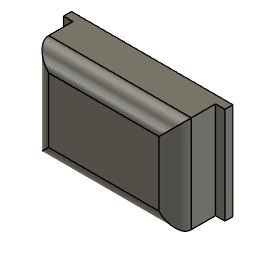
mds-0027 (Autodesk Fusion 360 archive; units mm, degrees)
design "Side-Button"
Autodesk Fusion 360 part; units mm, degrees
note: some values were not read from the file. Chosen so that the rebuilt part matches the saved one: which bodies a step acts on; which face or edge a step refers to. Set by a fixed rule: which sketch regions a step uses.
sketch "Sketch1" plane through (0, 0, 0) normal (0, 0, 1) x (1, 0, 0)
  line L0 (-30, 20) -> (-12.335, 20)
  line L1 (-12.335, 20) -> (-12.335, 8)
  line L2 (-12.335, 8) -> (-30, 8)
  line L3 (-30, 8) -> (-30, 20)
  dimension "d1" = 17.665
  dimension "d2" = 12
  constraint horizontal L0
  constraint vertical L1
  constraint horizontal L2
  constraint vertical L3
  measures "d1" distance of L0.start L0.end
  measures "d2" distance of L0.start L2.end
extrude "Extrude1" add sketch "Sketch1" along normal blind 6
fillet "Fillet1" radius 2 4 edges at (-21.1675, 20, 6) (-12.335, 14, 6) (-30, 14, 6) (-21.1675, 8, 6)
sketch "Sketch2" plane through (0, 0, 0) normal (0, 0, -1) x (-1, 0, 0)
  line L0 (12.335, 8) -> (30, 8)
  line L1 (30, 8) -> (30, 20)
  line L2 (30, 20) -> (12.335, 20)
  line L3 (12.335, 20) -> (12.335, 8)
  line L4 (11.1675, 20) -> (31.1675, 20)
  line L5 (11.1675, 8) -> (31.1675, 8)
  line L6 (31.1675, 20) -> (31.1675, 8)
  line L7 (11.1675, 8) -> (11.1675, 20)
  point P0 (21.1675, 20)
  point P1 (21.1675, 8)
  dimension "d7" = 20
  constraint midpoint L4 P0
  constraint coincident L2 P0
  constraint parallel L2 L4
  constraint midpoint L5 P1
  constraint coincident L0 P1
  constraint perpendicular L1 L5
  constraint perpendicular L5 L6
  constraint perpendicular L4 L7
  measures "d7" distance of L4.start L4.end
extrude "Extrude2" add sketch "Sketch2" against normal blind 1 contours L3 L4 L5 L7 | L1 L4 L5 L6

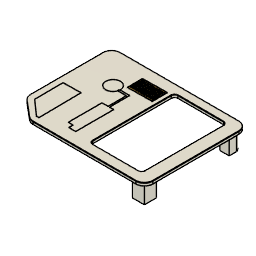
design "Lid" references "Main Casing"
Autodesk Fusion 360 part; units mm, degrees
other "Sketch2"
sketch "sketch 220" plane through (0, 0, 0) normal (0, 1, 0) x (1, 0, 0)
  line L0 (47.500001, 39.500001) -> (45.536455, 39.500001)
  line L1 (52.536455, 32.500001) -> (52.536455, 33)
  line L2 (45.536455, 39.500001) -> (-52.546208, 39.500001)
  line L3 (-59.546208, 32.500001) -> (-59.546208, -27.533953)
  line L4 (-39.426481, -45.554934) -> (45.536455, -45.554934)
  line L5 (52.536455, -38.554934) -> (52.536455, 32.500001)
  arc A0 (-52.546208, 39.500001) -> (-59.546208, 32.500001) centre (-52.546208, 32.500001) ccw
  arc A1 (45.536455, -45.554934) -> (52.536455, -38.554934) centre (45.536455, -38.554934) ccw
  line L6 (-57.048651, -32.893804) -> (-43.928925, -43.914786)
  arc A2 (-43.928925, -43.914786) -> (-39.426481, -45.554934) centre (-39.426481, -38.554934) ccw
  arc A3 (-59.546208, -27.533953) -> (-57.048651, -32.893804) centre (-52.546208, -27.533953) ccw
  line L7 (-57.046208, 32.500001) -> (-57.046208, -27.533953)
  arc A4 (-57.046208, -27.533953) -> (-55.440635, -30.979572) centre (-52.546208, -27.533953) ccw
  line L8 (-55.440635, -30.979572) -> (-42.320909, -42.000553)
  arc A5 (-42.320909, -42.000553) -> (-39.426481, -43.054934) centre (-39.426481, -38.554934) ccw
  line L9 (-39.426481, -43.054934) -> (45.536455, -43.054934)
  arc A6 (45.536455, -43.054934) -> (50.036455, -38.554934) centre (45.536455, -38.554934) ccw
  line L10 (50.036455, -38.554934) -> (50.036455, 32.500001)
  line L11 (45.536455, 37.000001) -> (-52.546208, 37.000001)
  arc A7 (-52.546208, 37.000001) -> (-57.046208, 32.500001) centre (-52.546208, 32.500001) ccw
  arc A8 (52.536455, 32.500001) -> (45.536455, 39.500001) centre (45.536455, 32.500001) ccw
  arc A9 (50.036455, 32.500001) -> (45.536455, 37.000001) centre (45.536455, 32.500001) ccw
extrude "Extrude1" add sketch "sketch 220" along normal blind 2 contours L2 L3 L4 L5 A0 A1 L6 A2 A3 A8 | L7 A4 L8 A5 L9 A6 L10 L11 A7 A9 picked at (-19.851987, 38.666667) picked at (-15.478745, 10.315022) makes body 1
sketch "Sketch2 (1)" plane through (0, 2, 0) normal (0, 1, 0) x (-1, 0, 0)
  arc A0 (59.546208, 27.533953) -> (57.048651, 32.893804) centre (52.546208, 27.533953) ccw
  line L0 (57.048651, 32.893804) -> (43.928925, 43.914786)
  arc A1 (43.928925, 43.914786) -> (39.426481, 45.554934) centre (39.426481, 38.554934) ccw
  line L1 (39.426481, 45.554934) -> (-45.536455, 45.554934)
  arc A2 (-45.536455, 45.554934) -> (-52.536455, 38.554934) centre (-45.536455, 38.554934) ccw
  line L2 (-52.536455, 38.554934) -> (-52.536455, -32.500001)
  line L3 (-45.536455, -39.500001) -> (52.546208, -39.500001)
  arc A3 (52.546208, -39.500001) -> (59.546208, -32.500001) centre (52.546208, -32.500001) ccw
  line L4 (59.546208, -32.500001) -> (59.546208, 27.533953)
  line L5 (39.853527, 5.449503) -> (39.426481, 40.606798)
  line L6 (39.426481, 40.606798) -> (41.485756, 40.631812)
  line L7 (41.485756, 40.631812) -> (54.299999, 29.299999)
  line L8 (54.299999, 29.299999) -> (54.499999, 5.7)
  line L9 (54.499999, 5.7) -> (39.853527, 5.449503)
  line L10 (4.205552, -17.763056) -> (24.5, -17.5)
  line L11 (24.5, -17.5) -> (24.662478, -30.03501)
  line L12 (24.662478, -30.03501) -> (4.288926, -30.299091)
  line L13 (4.288926, -30.299091) -> (4.205552, -17.763056)
  arc A4 (-52.536455, -32.500001) -> (-45.536455, -39.500001) centre (-45.536455, -32.500001) ccw
  constraint perpendicular L5 L6
  constraint perpendicular L10 L11
  constraint perpendicular L11 L12
extrude "Extrude2" add sketch "Sketch2 (1)" along normal blind 0.5 contours L5 L6 L7 L8 L9 | L10 L11 L12 L13 picked at (44.526669, 25.118767) picked at (11.052319, -26.032386) bodies 1
sketch "Sketch2" plane through (0, 2, 0) normal (0, 1, 0) x (-1, 0, 0)
  line L0 (54.499999, 5.7) -> (39.853527, 5.449503)
  line L1 (39.853527, 5.449503) -> (39.426481, 40.606798)
  line L2 (39.426481, 40.606798) -> (41.485756, 40.631812)
  line L3 (41.485756, 40.631812) -> (54.299999, 29.299999)
  line L4 (54.299999, 29.299999) -> (54.499999, 5.7)
  line L5 (4.288926, -30.299091) -> (4.205552, -17.763056)
  line L6 (4.205552, -17.763056) -> (24.5, -17.5)
  line L7 (24.5, -17.5) -> (24.662478, -30.03501)
  line L8 (24.662478, -30.03501) -> (4.288926, -30.299091)
  arc A0 (59.546208, 27.533953) -> (57.048651, 32.893804) centre (52.546208, 27.533953) ccw
  line L9 (57.048651, 32.893804) -> (43.928925, 43.914786)
  arc A1 (43.928925, 43.914786) -> (39.426481, 45.554934) centre (39.426481, 38.554934) ccw
  line L10 (39.426481, 45.554934) -> (-45.536455, 45.554934)
  arc A2 (-45.536455, 45.554934) -> (-52.536455, 38.554934) centre (-45.536455, 38.554934) ccw
  line L11 (-52.536455, 38.554934) -> (-52.536455, -32.500001)
  line L12 (-45.536455, -39.500001) -> (52.546208, -39.500001)
  arc A3 (52.546208, -39.500001) -> (59.546208, -32.500001) centre (52.546208, -32.500001) ccw
  line L13 (59.546208, -32.500001) -> (59.546208, 27.533953)
  line L14 (-42.294458, -30.655503) -> (3.504877, -30.655503)
  line L15 (3.504877, -30.655503) -> (3.504877, 35.741851)
  line L16 (3.504877, 35.741851) -> (-42.294458, 35.741851)
  line L17 (-42.294458, 35.741851) -> (-42.294458, -30.655503)
  line L18 (11, 17) -> (3.504877, 17)
  line L19 (3.504877, 17) -> (3.504877, 31.823372)
  line L20 (3.504877, 31.823372) -> (11, 31.823372)
  line L21 (11, 31.823372) -> (11, 17)
  line L22 (24, 4) -> (14.343, 4)
  line L23 (14.343, 4) -> (14.343, 31.823372)
  line L24 (14.343, 31.823372) -> (24, 31.823372)
  line L25 (24, 31.823372) -> (24, 4)
  line L26 (20.047669, 31.823372) -> (14.343, 31.823372)
  line L27 (14.343, 31.823372) -> (14.343, 35.373002)
  line L28 (14.343, 35.373002) -> (20.047669, 35.373002)
  line L29 (20.047669, 35.373002) -> (20.047669, 31.823372)
  line L30 (19, 4) -> (17.792239, 4)
  line L31 (17.792239, 4) -> (17.792239, -12.601724)
  line L32 (17.792239, -12.601724) -> (19, -12.601724)
  line L33 (19, -12.601724) -> (19, 4)
  line L34 (19, -12.601724) -> (26.334489, -12.601724)
  line L35 (26.334489, -12.601724) -> (26.334489, -11.113985)
  line L36 (26.334489, -11.113985) -> (19, -11.113985)
  line L37 (19, -11.113985) -> (19, -12.601724)
  circle A4 centre (31.789244, -12.921514) radius 6.052195
  arc A5 (-52.536455, -32.500001) -> (-45.536455, -39.500001) centre (-45.536455, -32.500001) ccw
  constraint horizontal L14
  constraint vertical L15
  constraint horizontal L16
  constraint vertical L17
  constraint horizontal L18
  constraint vertical L19
  constraint horizontal L20
  constraint vertical L21
  constraint horizontal L22
  constraint vertical L23
  constraint horizontal L24
  constraint vertical L25
  constraint horizontal L26
  constraint vertical L27
  constraint horizontal L28
  constraint vertical L29
  constraint horizontal L30
  constraint vertical L31
  constraint horizontal L32
  constraint vertical L33
  constraint coincident L22 L30.start
  constraint horizontal L34
  constraint vertical L35
  constraint horizontal L36
  constraint vertical L37
extrude "Extrude3" add sketch "Sketch2" along normal blind 0.5 separate body contours L14 L15 L16 L17 L19 | L15 L18 L19 L20 L21 | L22 L23 L24 L25 L26 L30 | L22 L30 L31 L32 L33 L37 | L33 L34 L36 L37 A4 | L24 L26 L27 L28 L29 | L34 L35 L36 A4 picked at (-27.028013, 7.362116) picked at (8.501626, 26.882248) picked at (17.394302, 22.548915) picked at (18.194826, -6.571903) picked at (21.264404, -11.938213) picked at (18.146112, 33.006582) picked at (33.983321, -12.514669) makes body 2 at (-33.99295, 2, -12.93937) makes body 2 at (-16.244556, 2, 23.732125) makes body 3 at (27.028013, 2, 7.362116)
sketch "Sketch3" plane through (0, 2, 0) normal (0, 1, 0) x (-1, 0, 0)
  line L0 (54.499999, 5.7) -> (39.853527, 5.449503)
  line L1 (39.853527, 5.449503) -> (39.426481, 40.606798)
  line L2 (39.426481, 40.606798) -> (41.485756, 40.631812)
  line L3 (41.485756, 40.631812) -> (54.299999, 29.299999)
  line L4 (54.299999, 29.299999) -> (54.499999, 5.7)
  line L5 (4.288926, -30.299091) -> (4.205552, -17.763056)
  line L6 (4.205552, -17.763056) -> (24.5, -17.5)
  line L7 (24.5, -17.5) -> (24.662478, -30.03501)
  line L8 (24.662478, -30.03501) -> (4.288926, -30.299091)
  arc A0 (59.546208, 27.533953) -> (57.048651, 32.893804) centre (52.546208, 27.533953) ccw
  line L9 (57.048651, 32.893804) -> (43.928925, 43.914786)
  arc A1 (43.928925, 43.914786) -> (39.426481, 45.554934) centre (39.426481, 38.554934) ccw
  line L10 (39.426481, 45.554934) -> (-45.536455, 45.554934)
  arc A2 (-45.536455, 45.554934) -> (-52.536455, 38.554934) centre (-45.536455, 38.554934) ccw
  line L11 (-52.536455, 38.554934) -> (-52.536455, -32.500001)
  line L12 (-45.536455, -39.500001) -> (52.546208, -39.500001)
  arc A3 (52.546208, -39.500001) -> (59.546208, -32.500001) centre (52.546208, -32.500001) ccw
  line L13 (59.546208, -32.500001) -> (59.546208, 27.533953)
  line L14 (3.505741, -0.818006) -> (21.505741, -0.818006)
  line L15 (21.505741, -0.818006) -> (21.505741, 9)
  line L16 (21.505741, 9) -> (3.505741, 9)
  line L17 (3.505741, 9) -> (3.505741, -0.818006)
  circle A4 centre (26.7, 3.4) radius 7.710383
  circle A5 centre (26.7, 3.4) radius 3.809172
  line L18 (26.255748, -0.383177) -> (26.255748, -4.297574)
  line L19 (24.091779, 0.623857) -> (21.552371, -2.340375)
  line L20 (29.308222, 0.623857) -> (32.279495, -1.921583)
  line L21 (30.435008, 4.148002) -> (34.374015, 4.148002)
  line L22 (27.960024, 6.994736) -> (30.435008, 10.145348)
  line L23 (24.971982, 6.794663) -> (22.964993, 10.145348)
  line L24 (22.964986, 4.147965) -> (19.025983, 4.147965)
  arc A6 (-52.536455, -32.500001) -> (-45.536455, -39.500001) centre (-45.536455, -32.500001) ccw
  dimension "d7" = 18
  constraint horizontal L14
  constraint vertical L15
  constraint horizontal L16
  constraint vertical L17
  constraint concentric A4 A5
  constraint vertical L18
  constraint perpendicular L19 L20
  constraint horizontal L21
  constraint perpendicular L15 L24
extrude "Extrude4" add sketch "Sketch3" 1 faces at (0.634807, 2, 22.799559) along normal blind 0.5 separate body contours L14 L16 L17 A4 | L14 L15 A4 L24 | L14 L15 A4 A5 L19 L24 | L15 L16 A4 L24 | A4 A5 L18 L19 | L15 L16 A4 A5 L23 L24 | A4 A5 L18 L20 | A5 | A4 A5 L22 L23 | A4 A5 L20 L21 | A4 A5 L21 L22 picked at (8.679155, 4.109986) picked at (20.788323, 1.463096) picked at (22.002936, 1.945177) picked at (19.914302, 4.510346) picked at (25.912582, -2.949659) picked at (22.178116, 6.216434) picked at (26.810645, -2.995525) picked at (24.522142, 2.626677) picked at (23.970696, 9.184282) picked at (31.616215, -0.696826) picked at (33.002229, 4.498209) on bodies 1 makes body 4
sketch "Sketch4" plane through (0, 2.5, 0) normal (0, 1, 0) x (-1, 0, 0)
  line L0 (3.504877, 17) -> (11, 17)
  line L1 (11, 17) -> (11, 31.823372)
  line L2 (11, 31.823372) -> (3.504877, 31.823372)
sketch "Sketch6" plane through (0, 0, 0) normal (0, -1, 0) x (1, 0, 0)
  arc A0 (-57.048651, 32.893804) -> (-59.546208, 27.533953) centre (-52.546208, 27.533953) ccw
  line L0 (-59.546208, 27.533953) -> (-59.546208, -32.500001)
  arc A1 (-59.546208, -32.500001) -> (-52.546208, -39.500001) centre (-52.546208, -32.500001) ccw
  line L1 (-52.546208, -39.500001) -> (45.536455, -39.500001)
  line L2 (52.536455, -32.500001) -> (52.536455, 38.554934)
  arc A2 (52.536455, 38.554934) -> (45.536455, 45.554934) centre (45.536455, 38.554934) ccw
  line L3 (45.536455, 45.554934) -> (-39.426481, 45.554934)
  arc A3 (-39.426481, 45.554934) -> (-43.928925, 43.914786) centre (-39.426481, 38.554934) ccw
  line L4 (-43.928925, 43.914786) -> (-57.048651, 32.893804)
  arc A4 (45.536455, -37.000001) -> (50.036455, -32.500001) centre (45.536455, -32.500001) ccw
  line L5 (50.000001, -37.000001) -> (40.000001, -37.000001)
  line L6 (40.000001, -37.000001) -> (40.000001, -27.000001)
  line L7 (40.000001, -27.000001) -> (50.000001, -27.000001)
  line L8 (50.000001, -27.000001) -> (50.000001, -37.000001)
  line L9 (50.000001, 43.000001) -> (40.000001, 43.000001)
  line L10 (40.000001, 43.000001) -> (40.000001, 33.000001)
  line L11 (40.000001, 33.000001) -> (50.000001, 33.000001)
  line L12 (50.000001, 33.000001) -> (50.000001, 43.000001)
  line L13 (-57.000001, -37.000001) -> (-47.000001, -37.000001)
  line L14 (-47.000001, -37.000001) -> (-47.000001, -27.000001)
  line L15 (-47.000001, -27.000001) -> (-57.000001, -27.000001)
  line L16 (-57.000001, -27.000001) -> (-57.000001, -37.000001)
  circle A5 centre (45.536455, -32.500001) radius 1.5
  circle A6 centre (-52.546208, -32.500001) radius 1.5
  circle A7 centre (45.536455, 38.554934) radius 1.5
  arc A8 (45.536455, -39.500001) -> (52.536455, -32.500001) centre (45.536455, -32.500001) ccw
  line L17 (52.536455, -32.500001) -> (52.536455, 38.554934)
  arc A9 (52.536455, 38.554934) -> (45.536455, 45.554934) centre (45.536455, 38.554934) ccw
  line L18 (45.536455, 45.554934) -> (-39.426481, 45.554934)
  arc A10 (-39.426481, 45.554934) -> (-43.928925, 43.914786) centre (-39.426481, 38.554934) ccw
  line L19 (-43.928925, 43.914786) -> (-57.048651, 32.893804)
  arc A11 (-57.048651, 32.893804) -> (-59.546208, 27.533953) centre (-52.546208, 27.533953) ccw
  line L20 (-59.546208, 27.533953) -> (-59.546208, -32.500001)
  arc A12 (-59.546208, -32.500001) -> (-52.546208, -39.500001) centre (-52.546208, -32.500001) ccw
  line L21 (-52.546208, -39.500001) -> (45.536455, -39.500001)
  arc A13 (45.536455, -39.500001) -> (52.536455, -32.500001) centre (45.536455, -32.500001) ccw
  line L22 (50.036455, -32.500001) -> (50.036455, 38.554934)
  arc A14 (50.036455, 38.554934) -> (45.536455, 43.054934) centre (45.536455, 38.554934) ccw
  line L23 (45.536455, 43.054934) -> (-39.426481, 43.054934)
  arc A15 (-39.426481, 43.054934) -> (-42.320909, 42.000553) centre (-39.426481, 38.554934) ccw
  line L24 (-42.320909, 42.000553) -> (-55.440635, 30.979572)
  arc A16 (-55.440635, 30.979572) -> (-57.046208, 27.533953) centre (-52.546208, 27.533953) ccw
  line L25 (-57.046208, 27.533953) -> (-57.046208, -32.500001)
  arc A17 (-57.046208, -32.500001) -> (-52.546208, -37.000001) centre (-52.546208, -32.500001) ccw
  line L26 (-52.546208, -37.000001) -> (45.536455, -37.000001)
  arc A18 (45.536455, -37.000001) -> (50.036455, -32.500001) centre (45.536455, -32.500001) ccw
  dimension "d21" = 0
  dimension "d22" = -2.5
  dimension "d23" = 10
  dimension "d24" = 10
  dimension "d25" = 10
  dimension "d26" = 10
  dimension "d27" = 10
  dimension "d28" = 10
  dimension "d29" = 3
  dimension "d30" = 3
  dimension "d31" = 3
  constraint horizontal L5
  constraint vertical L6
  constraint horizontal L7
  constraint vertical L8
  constraint horizontal L9
  constraint vertical L10
  constraint horizontal L11
  constraint vertical L12
  constraint horizontal L13
  constraint vertical L14
  constraint horizontal L15
  constraint vertical L16
  constraint concentric A1 A6
  constraint concentric A2 A7
  measures "d21" distance of L1
  measures "d29" diameter of A5
  measures "d30" diameter of A6
  measures "d31" diameter of A7
extrude "Extrude6" add sketch "Sketch6" along normal blind 14 contours A4 L5 L6 L7 L8 L26 A18 | L13 L14 L15 L16 A17 L26 | L13 L16 A17 | L9 L12 A14 | L9 L10 L11 L12 A14 picked at (41.35107, -32.092146) picked at (-48.354321, -32.092146) picked at (-56.145994, -36.116652) picked at (49.170703, 42.121578) picked at (45.141454, 34.353043) bodies 1
sketch "Sketch8" plane through (0, 2.5, 0) normal (0, 1, 0) x (-1, 0, 0)
  line L0 (-42.280199, -30.654372) -> (-42.280199, 35.233479)
  line L1 (-42.280199, -30.160446) -> (-42.280199, 37.539554)
  line L2 (-39.480199, -32.960446) -> (-1.780199, -32.960446)
  line L3 (1.019801, -32.960446) -> (1.019801, 37.539554)
  line L4 (-1.780199, 37.539554) -> (-39.480199, 37.539554)
  line L5 (-42.280199, 34.739554) -> (-42.280199, -32.960446)
  line L6 (-42.280199, -32.960446) -> (-39.780199, -32.960446)
  line L7 (-39.780199, -32.960446) -> (-39.780199, -30.460446)
  line L8 (-39.780199, -30.460446) -> (-42.280199, -30.460446)
  line L9 (-42.280199, -30.460446) -> (-42.280199, -32.960446)
  circle A0 centre (-39.780199, -30.460446) radius 1.5
  line L10 (1.019801, -32.960446) -> (-1.480199, -32.960446)
  line L11 (-1.480199, -32.960446) -> (-1.480199, -30.460446)
  line L12 (-1.480199, -30.460446) -> (1.019801, -30.460446)
  line L13 (1.019801, -30.460446) -> (1.019801, -30.160446)
  circle A1 centre (-1.480199, -30.460446) radius 1.5
  line L14 (1.019801, 37.539554) -> (-1.480199, 37.539554)
  line L15 (-1.480199, 37.539554) -> (-1.480199, 35.039554)
  line L16 (-1.480199, 35.039554) -> (1.019801, 35.039554)
  line L17 (1.019801, 35.039554) -> (1.019801, 34.739554)
  circle A2 centre (-1.480199, 35.039554) radius 1.5
  line L18 (-42.280199, 37.539554) -> (-39.780199, 37.539554)
  line L19 (-39.780199, 37.539554) -> (-39.780199, 35.039554)
  line L20 (-39.780199, 35.039554) -> (-42.280199, 35.039554)
  line L21 (-42.280199, 35.039554) -> (-42.280199, 37.539554)
  circle A3 centre (-39.780199, 35.039554) radius 1.5
  arc A4 (-1.780199, -32.960446) -> (1.019801, -30.160446) centre (-1.780199, -30.160446) ccw
  arc A5 (-42.280199, -30.160446) -> (-39.480199, -32.960446) centre (-39.480199, -30.160446) ccw
  arc A6 (-39.480199, 37.539554) -> (-42.280199, 34.739554) centre (-39.480199, 34.739554) ccw
  arc A7 (1.019801, 34.739554) -> (-1.780199, 37.539554) centre (-1.780199, 34.739554) ccw
  point P0 (-42.280199, 2.289554)
  point P1 (-42.280199, 37.539554)
  dimension "d34" = 70.5
  dimension "d35" = 43.3
  dimension "d36" = 70.5
  dimension "d46" = 2.5
  dimension "d47" = 2.5
  dimension "d48" = 3
  dimension "d49" = 2.5
  dimension "d50" = 2.5
  dimension "d51" = 3
  dimension "d52" = 2.5
  dimension "d53" = 2.5
  dimension "d54" = 3
  dimension "d55" = 2.5
  dimension "d56" = 2.5
  dimension "d57" = 3
  dimension "d58" = 2.8
  constraint vertical L0
  constraint parallel L0 L1
  constraint horizontal L2
  constraint vertical L3
  constraint horizontal L4
  constraint vertical L5
  constraint horizontal L6
  constraint vertical L7
  constraint horizontal L8
  constraint vertical L9
  constraint horizontal L10
  constraint vertical L11
  constraint horizontal L12
  constraint vertical L13
  constraint horizontal L14
  constraint vertical L15
  constraint horizontal L16
  constraint vertical L17
  constraint horizontal L18
  constraint vertical L19
  constraint horizontal L20
  constraint vertical L21
  constraint tangent L13 A4
  constraint tangent L2 A4
  constraint tangent L1 A5
  constraint tangent L2 A5
  constraint equal A4 A5
  constraint tangent L5 A6
  constraint tangent L4 A6
  constraint equal A4 A6
  constraint tangent L17 A7
  constraint tangent L4 A7
  constraint equal A4 A7
  measures "d48" diameter of A0
  measures "d51" diameter of A1
  measures "d54" diameter of A2
  measures "d57" diameter of A3
  measures "d58" radius of A4
extrude "Extrude7" cut sketch "Sketch8" against normal blind 20 contours L0 L1 L2 L3 L4 L5 L7 L8 A0 L11 L12 A1 L15 L16 A2 L19 L20 A3 A4 A5 A6 A7 | L7 L8 A0 A5 | L7 L8 A0 | L7 L8 A0 | L19 L20 A3 A6 | L19 L20 A3 | L19 L20 A3 | L11 L12 A1 A4 | L11 L12 A1 | L11 L12 A1 | L15 L16 A2 A7 | L15 L16 A2 | L15 L16 A2 picked at (-26.749231, -8.186152) picked at (-41.914081, -30.584983) picked at (-40.774614, -30.385925) picked at (-39.992223, -31.435104) picked at (-39.904736, 37.173436) picked at (-40.5787, 35.637304) picked at (-40.774614, 34.965033) picked at (-1.355662, -32.594329) picked at (-2.477189, -30.484921) picked at (-0.774894, -31.165751) picked at (-1.355662, 37.173436) picked at (-0.485288, 35.110711) picked at (-2.322763, 34.506006) bodies 1 3 4 makes body 5 at (42.294458, 2.166667, 13.6094)
sketch "Sketch9" plane through (0, 2.5, 0) normal (0, 1, 0) x (-1, 0, 0)
  line L0 (-1.780199, -32.960446) -> (-39.480199, -32.960446)
  line L1 (-42.280199, -30.160446) -> (-42.280199, 34.739554)
  line L2 (-39.480199, 37.539554) -> (-1.780199, 37.539554)
  line L3 (1.019801, 34.739554) -> (1.019801, -30.160446)
  line L4 (54.499999, 5.7) -> (39.853527, 5.449503)
  line L5 (39.853527, 5.449503) -> (39.426481, 40.606798)
  line L6 (39.426481, 40.606798) -> (41.485756, 40.631812)
  line L7 (41.485756, 40.631812) -> (54.299999, 29.299999)
  line L8 (54.299999, 29.299999) -> (54.499999, 5.7)
  line L9 (4.288926, -30.299091) -> (4.205552, -17.763056)
  line L10 (4.205552, -17.763056) -> (24.5, -17.5)
  line L11 (24.5, -17.5) -> (24.662478, -30.03501)
  line L12 (24.662478, -30.03501) -> (4.288926, -30.299091)
  arc A0 (59.546208, 27.533953) -> (57.048651, 32.893804) centre (52.546208, 27.533953) ccw
  line L13 (57.048651, 32.893804) -> (43.928925, 43.914786)
  arc A1 (43.928925, 43.914786) -> (39.426481, 45.554934) centre (39.426481, 38.554934) ccw
  line L14 (39.426481, 45.554934) -> (-45.536455, 45.554934)
  arc A2 (-45.536455, 45.554934) -> (-52.536455, 38.554934) centre (-45.536455, 38.554934) ccw
  line L15 (-52.536455, 38.554934) -> (-52.536455, -32.500001)
  line L16 (-45.536455, -39.500001) -> (52.546208, -39.500001)
  arc A3 (52.546208, -39.500001) -> (59.546208, -32.500001) centre (52.546208, -32.500001) ccw
  line L17 (59.546208, -32.500001) -> (59.546208, 27.533953)
  arc A4 (-52.536455, -32.500001) -> (-45.536455, -39.500001) centre (-45.536455, -32.500001) ccw
  arc A5 (-1.780199, -32.960446) -> (1.019801, -30.160446) centre (-1.780199, -30.160446) ccw
  arc A6 (-42.280199, -30.160446) -> (-39.480199, -32.960446) centre (-39.480199, -30.160446) ccw
  arc A7 (-39.480199, 37.539554) -> (-42.280199, 34.739554) centre (-39.480199, 34.739554) ccw
  arc A8 (1.019801, 34.739554) -> (-1.780199, 37.539554) centre (-1.780199, 34.739554) ccw
sketch "Sketch10" plane through (0, 0, 0) normal (0, -1, 0) x (1, 0, 0)
  line L0 (-57.000001, -27.000001) -> (-47.000001, -27.000001)
  line L1 (-47.000001, -27.000001) -> (-47.000001, -37.000001)
  line L2 (-47.000001, -37.000001) -> (-57.000001, -37.000001)
  line L3 (-57.000001, -37.000001) -> (-57.000001, -27.000001)
  line L4 (39.480199, -32.960446) -> (1.780199, -32.960446)
  line L5 (-1.019801, -30.160446) -> (-1.019801, 34.739554)
  line L6 (1.780199, 37.539554) -> (39.480199, 37.539554)
  line L7 (40.000001, 37.490882) -> (40.000001, 43.000001)
  line L8 (40.000001, 43.000001) -> (50.000001, 43.000001)
  line L9 (50.000001, 43.000001) -> (50.000001, 33.000001)
  line L10 (50.000001, 33.000001) -> (42.280199, 33.000001)
  line L11 (42.280199, 33.000001) -> (42.280199, -27.000001)
  line L12 (42.280199, -27.000001) -> (50.000001, -27.000001)
  line L13 (50.000001, -27.000001) -> (50.000001, -33.071626)
  arc A0 (45.536455, -37.000001) -> (50.000001, -33.071626) centre (45.536455, -32.500001) ccw
  line L14 (45.536455, -37.000001) -> (40.000001, -37.000001)
  line L15 (40.000001, -37.000001) -> (40.000001, -32.911774)
  arc A1 (45.536455, -39.500001) -> (52.536455, -32.500001) centre (45.536455, -32.500001) ccw
  line L16 (52.536455, -32.500001) -> (52.536455, 38.554934)
  arc A2 (52.536455, 38.554934) -> (45.536455, 45.554934) centre (45.536455, 38.554934) ccw
  line L17 (45.536455, 45.554934) -> (-39.426481, 45.554934)
  arc A3 (-39.426481, 45.554934) -> (-43.928925, 43.914786) centre (-39.426481, 38.554934) ccw
  line L18 (-43.928925, 43.914786) -> (-57.048651, 32.893804)
  arc A4 (-57.048651, 32.893804) -> (-59.546208, 27.533953) centre (-52.546208, 27.533953) ccw
  line L19 (-59.546208, 27.533953) -> (-59.546208, -32.500001)
  arc A5 (-59.546208, -32.500001) -> (-52.546208, -39.500001) centre (-52.546208, -32.500001) ccw
  line L20 (-52.546208, -39.500001) -> (45.536455, -39.500001)
  circle A6 centre (-52.546208, -32.500001) radius 1.5
  circle A7 centre (45.536455, 38.554934) radius 1.5
  circle A8 centre (45.536455, -32.500001) radius 1.5
  arc A9 (40.000001, 37.490882) -> (39.480199, 37.539554) centre (39.480199, 34.739554) ccw
  arc A10 (39.480199, -32.960446) -> (40.000001, -32.911774) centre (39.480199, -30.160446) ccw
  arc A11 (-1.019801, -30.160446) -> (1.780199, -32.960446) centre (1.780199, -30.160446) ccw
  arc A12 (1.780199, 37.539554) -> (-1.019801, 34.739554) centre (1.780199, 34.739554) ccw
  dimension "d41" = 3
  dimension "d42" = 3
  dimension "d43" = 3
  constraint concentric A5 A6
  constraint concentric A2 A7
  constraint concentric A0 A8
  measures "d41" diameter of A6
  measures "d42" diameter of A7
  measures "d43" diameter of A8
extrude "Extrude9" add sketch "Sketch10" along normal blind 5 contours A6 | A7 | A8 picked at (-52.734463, -33.039959) picked at (46.253391, 38.480413) picked at (45.348199, -33.039959) bodies 1
sketch "Sketch11" plane through (0, 2.5, 0) normal (0, 1, 0) x (-1, 0, 0)
  line L0 (-39.480199, 37.539554) -> (-1.780199, 37.539554)
  arc A0 (1.019801, 34.739554) -> (-1.780199, 37.539554) centre (-1.780199, 34.739554) ccw
  line L1 (1.019801, 34.739554) -> (1.019801, -30.160446)
  arc A1 (-1.780199, -32.960446) -> (1.019801, -30.160446) centre (-1.780199, -30.160446) ccw
  line L2 (-1.780199, -32.960446) -> (-39.480199, -32.960446)
  arc A2 (-42.280199, -30.160446) -> (-39.480199, -32.960446) centre (-39.480199, -30.160446) ccw
  line L3 (-42.280199, -30.160446) -> (-42.280199, 34.739554)
  arc A3 (-39.480199, 37.539554) -> (-42.280199, 34.739554) centre (-39.480199, 34.739554) ccw
  line L4 (54.499999, 5.7) -> (39.853527, 5.449503)
  line L5 (39.853527, 5.449503) -> (39.426481, 40.606798)
  line L6 (39.426481, 40.606798) -> (41.485756, 40.631812)
  line L7 (41.485756, 40.631812) -> (54.299999, 29.299999)
  line L8 (54.299999, 29.299999) -> (54.499999, 5.7)
  line L9 (4.288926, -30.299091) -> (4.205552, -17.763056)
  line L10 (4.205552, -17.763056) -> (24.5, -17.5)
  line L11 (24.5, -17.5) -> (24.662478, -30.03501)
  line L12 (24.662478, -30.03501) -> (4.288926, -30.299091)
  arc A4 (-52.536455, -32.500001) -> (-45.536455, -39.500001) centre (-45.536455, -32.500001) ccw
  line L13 (-45.536455, -39.500001) -> (52.546208, -39.500001)
  arc A5 (52.546208, -39.500001) -> (59.546208, -32.500001) centre (52.546208, -32.500001) ccw
  line L14 (59.546208, -32.500001) -> (59.546208, 27.533953)
  arc A6 (59.546208, 27.533953) -> (57.048651, 32.893804) centre (52.546208, 27.533953) ccw
  line L15 (57.048651, 32.893804) -> (43.928925, 43.914786)
  arc A7 (43.928925, 43.914786) -> (39.426481, 45.554934) centre (39.426481, 38.554934) ccw
  line L16 (39.426481, 45.554934) -> (-45.536455, 45.554934)
  arc A8 (-45.536455, 45.554934) -> (-52.536455, 38.554934) centre (-45.536455, 38.554934) ccw
  line L17 (-52.536455, 38.554934) -> (-52.536455, -32.500001)
  line L18 (24.662478, -30.03501) -> (4.205552, -30.03501)
  line L19 (4.205552, -30.03501) -> (4.205552, -17.763056)
  line L20 (4.205552, -17.763056) -> (24.662478, -17.763056)
  line L21 (24.662478, -17.763056) -> (24.662478, -30.03501)
  circle A9 centre (23.461462, -28.471271) radius 0.75
  circle A10 centre (21.825098, -28.471271) radius 0.75
  circle A11 centre (20.188735, -28.471271) radius 0.75
  circle A12 centre (18.552371, -28.471271) radius 0.75
  circle A13 centre (16.916007, -28.471271) radius 0.75
  circle A14 centre (15.279644, -28.471271) radius 0.75
  circle A15 centre (13.64328, -28.471271) radius 0.75
  circle A16 centre (12.006916, -28.471271) radius 0.75
  circle A17 centre (10.370553, -28.471271) radius 0.75
  circle A18 centre (8.734189, -28.471271) radius 0.75
  circle A19 centre (7.097826, -28.471271) radius 0.75
  circle A20 centre (5.461462, -28.471271) radius 0.75
  circle A21 centre (23.461462, -26.671271) radius 0.75
  circle A22 centre (21.825098, -26.671271) radius 0.75
  circle A23 centre (20.188735, -26.671271) radius 0.75
  circle A24 centre (18.552371, -26.671271) radius 0.75
  circle A25 centre (16.916007, -26.671271) radius 0.75
  circle A26 centre (15.279644, -26.671271) radius 0.75
  circle A27 centre (13.64328, -26.671271) radius 0.75
  circle A28 centre (12.006916, -26.671271) radius 0.75
  circle A29 centre (10.370553, -26.671271) radius 0.75
  circle A30 centre (8.734189, -26.671271) radius 0.75
  circle A31 centre (7.097826, -26.671271) radius 0.75
  circle A32 centre (5.461462, -26.671271) radius 0.75
  circle A33 centre (23.461462, -24.871271) radius 0.75
  circle A34 centre (21.825098, -24.871271) radius 0.75
  circle A35 centre (20.188735, -24.871271) radius 0.75
  circle A36 centre (18.552371, -24.871271) radius 0.75
  circle A37 centre (16.916007, -24.871271) radius 0.75
  circle A38 centre (15.279644, -24.871271) radius 0.75
  circle A39 centre (13.64328, -24.871271) radius 0.75
  circle A40 centre (12.006916, -24.871271) radius 0.75
  circle A41 centre (10.370553, -24.871271) radius 0.75
  circle A42 centre (8.734189, -24.871271) radius 0.75
  circle A43 centre (7.097826, -24.871271) radius 0.75
  circle A44 centre (5.461462, -24.871271) radius 0.75
  circle A45 centre (23.461462, -23.071271) radius 0.75
  circle A46 centre (21.825098, -23.071271) radius 0.75
  circle A47 centre (20.188735, -23.071271) radius 0.75
  circle A48 centre (18.552371, -23.071271) radius 0.75
  circle A49 centre (16.916007, -23.071271) radius 0.75
  circle A50 centre (15.279644, -23.071271) radius 0.75
  circle A51 centre (13.64328, -23.071271) radius 0.75
  circle A52 centre (12.006916, -23.071271) radius 0.75
  circle A53 centre (10.370553, -23.071271) radius 0.75
  circle A54 centre (8.734189, -23.071271) radius 0.75
  circle A55 centre (7.097826, -23.071271) radius 0.75
  circle A56 centre (5.461462, -23.071271) radius 0.75
  circle A57 centre (23.461462, -21.271271) radius 0.75
  circle A58 centre (21.825098, -21.271271) radius 0.75
  circle A59 centre (20.188735, -21.271271) radius 0.75
  circle A60 centre (18.552371, -21.271271) radius 0.75
  circle A61 centre (16.916007, -21.271271) radius 0.75
  circle A62 centre (15.279644, -21.271271) radius 0.75
  circle A63 centre (13.64328, -21.271271) radius 0.75
  circle A64 centre (12.006916, -21.271271) radius 0.75
  circle A65 centre (10.370553, -21.271271) radius 0.75
  circle A66 centre (8.734189, -21.271271) radius 0.75
  circle A67 centre (7.097826, -21.271271) radius 0.75
  circle A68 centre (5.461462, -21.271271) radius 0.75
  circle A69 centre (23.461462, -19.471271) radius 0.75
  circle A70 centre (21.825098, -19.471271) radius 0.75
  circle A71 centre (20.188735, -19.471271) radius 0.75
  circle A72 centre (18.552371, -19.471271) radius 0.75
  circle A73 centre (16.916007, -19.471271) radius 0.75
  circle A74 centre (15.279644, -19.471271) radius 0.75
  circle A75 centre (13.64328, -19.471271) radius 0.75
  circle A76 centre (12.006916, -19.471271) radius 0.75
  circle A77 centre (10.370553, -19.471271) radius 0.75
  circle A78 centre (8.734189, -19.471271) radius 0.75
  circle A79 centre (7.097826, -19.471271) radius 0.75
  circle A80 centre (5.461462, -19.471271) radius 0.75
  dimension "d59" = 1.5
  dimension "d62" = -18
  dimension "d63" = 9
  constraint horizontal L18
  constraint vertical L19
  constraint horizontal L20
  constraint vertical L21
  measures "d59" diameter of A9
extrude "Extrude10" cut sketch "Sketch11" against normal blind 4 contours A9 | A10 | A11 | A12 | A13 | A14 | A15 | A16 | A17 | A18 | A19 | A20 | A21 | A22 | A23 | A24 | A25 | A26 | A27 | A28 | A29 | A30 | A31 | A32 | A33 | A34 | A35 | A36 | A37 | A38 | A39 | A40 | A41 | A42 | A43 | A44 | A45 | A46 | A47 | A48 | A49 | A50 | A51 | A52 | A53 | A54 | A55 | A56 | A57 | A58 | A59 | A60 | A61 | A62 | A63 | A64 | A65 | A66 | A67 | A68 | A69 | A70 | A71 | A72 | A73 | A74 | A75 | A76 | A77 | A78 | A79 | A80 picked at (23.370127, -28.216526) picked at (21.733763, -28.216526) picked at (20.097399, -28.216526) picked at (18.461036, -28.216526) picked at (16.824672, -28.216526) picked at (14.926119, -28.601088) picked at (13.289755, -28.601088) picked at (11.653391, -28.601088) picked at (10.017028, -28.601088) picked at (8.527629, -28.612101) picked at (6.972826, -28.254765) picked at (5.586462, -28.687778) picked at (23.552797, -26.90399) picked at (21.916434, -26.90399) picked at (20.28007, -26.90399) picked at (18.643706, -26.90399) picked at (17.007343, -26.90399) picked at (15.370979, -26.438553) picked at (13.734615, -26.438553) picked at (12.098252, -26.438553) picked at (10.461888, -26.438553) picked at (8.578317, -26.475813) picked at (6.972826, -26.454765) picked at (5.586462, -26.887778) picked at (23.552797, -25.10399) picked at (21.916434, -25.10399) picked at (20.28007, -25.10399) picked at (18.643706, -25.10399) picked at (17.007343, -25.10399) picked at (15.370979, -24.638553) picked at (13.734615, -24.638553) picked at (12.098252, -24.638553) picked at (10.461888, -24.638553) picked at (8.578317, -24.675813) picked at (6.972826, -24.654765) picked at (5.586462, -25.087778) picked at (23.552797, -23.30399) picked at (21.916434, -23.30399) picked at (20.28007, -23.30399) picked at (18.643706, -23.30399) picked at (17.007343, -23.30399) picked at (15.370979, -22.838553) picked at (13.734615, -22.838553) picked at (12.098252, -22.838553) picked at (10.461888, -22.838553) picked at (8.578317, -22.875813) picked at (6.972826, -22.854765) picked at (5.586462, -23.287778) picked at (23.552797, -21.50399) picked at (21.916434, -21.50399) picked at (20.28007, -21.50399) picked at (18.643706, -21.50399) picked at (17.007343, -21.50399) picked at (15.370979, -21.038553) picked at (13.734615, -21.038553) picked at (12.098252, -21.038553) picked at (10.461888, -21.038553) picked at (8.578317, -21.075813) picked at (6.972826, -21.054765) picked at (5.586462, -21.487778) picked at (23.370127, -19.216526) picked at (21.733763, -19.216526) picked at (20.097399, -19.216526) picked at (18.461036, -19.216526) picked at (16.824672, -19.216526) picked at (14.926119, -19.601088) picked at (13.289755, -19.601088) picked at (11.653391, -19.601088) picked at (10.017028, -19.601088) picked at (8.527629, -19.612101) picked at (6.972826, -19.254765) picked at (5.586462, -19.687778) bodies 1
hidden bodies 3
